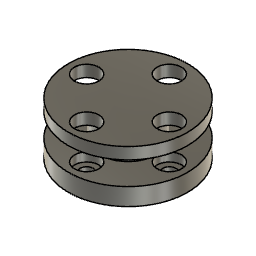
Pulley (Autodesk Fusion 360 design; units mm, degrees)
Autodesk Fusion 360 part; units mm, degrees
sketch "Sketch1" plane through (0, 0, 0) normal (0, 0, 1) x (1, 0, 0)
  circle A0 centre (0, 0) radius 10.3
  dimension "d1" = 20.6
  constraint coincident A0.centre origin
  measures "d1" diameter of A0
extrude "Extrude1" add sketch "Sketch1" along normal blind 3
sketch "Sketch2" plane through (0, 0, 3) normal (0, 0, 1) x (-1, 0, 0)
  circle A0 centre (0, 0) radius 10.3
  circle A1 centre (0, 0) radius 5
  dimension "d4" = 10
  constraint coincident A0.centre A1.centre
  measures "d4" diameter of A1
extrude "Extrude2" add sketch "Sketch2" along normal blind 4 contours A1
sketch "Sketch3" plane through (0, 0, 7) normal (0, 0, 1) x (-1, 0, 0)
  circle A0 centre (0, 0) radius 5
  circle A1 centre (0, 0) radius 10.3
  dimension "d7" = 20.6
  constraint coincident A0.centre A1.centre
  measures "d7" diameter of A1
extrude "Extrude3" add sketch "Sketch3" along normal blind 2 contours A0 | A1
sketch "Sketch4" plane through (0, 0, 9) normal (0, 0, 1) x (-1, 0, 0)
  circle A0 centre (0, 0) radius 10.3
  circle A1 centre (-7.15, 0) radius 1.1
  line L0 (0, 0) -> (-7.15, 0)
  dimension "d10" = 2.2
  dimension "d23" = 7.15
  constraint coincident A0.centre L0.start
  constraint horizontal L0
  constraint coincident A1.centre L0.end
  measures "d10" diameter of A1
  measures "d23" distance of A0.centre A1.centre
extrude "Extrude4" cut sketch "Sketch4" against normal blind 9 contours A1
pattern_circular "C-Pattern1" count 4 over 360 about axis through (0, 0, 7) along (0, 0, 1) of "Extrude4"
sketch "Sketch5" plane through (0, 0, 9) normal (0, 0, 1) x (-1, 0, 0)
  circle A0 centre (0, 7.15) radius 1.1
  circle A1 centre (7.15, 0) radius 1.1
  circle A2 centre (0, -7.15) radius 1.1
  circle A3 centre (-7.15, 0) radius 1.1
  circle A4 centre (0, 0) radius 10.3
  circle A5 centre (0, 7.15) radius 2.1
  dimension "d19" = 4.2
  constraint concentric A0 A5
  measures "d19" diameter of A5
extrude "Extrude5" cut sketch "Sketch5" against normal blind 7.5 contours A5
pattern_circular "C-Pattern2" count 4 over 360 about axis through (0, 0, 3) along (0, 0, 1) of "Extrude5"
hole "Hole1" at (5, 0, 4.7624) direction (-1, 0, 0) diameter 2 depth 10 tip angle 180
